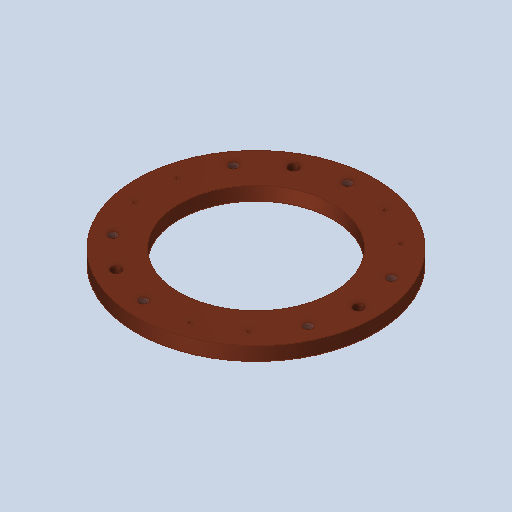
# Autodesk Inventor part: CentralRing-2023-1
Saved by Autodesk Inventor 2026 (Build 300175050, 175E)
## iProperties
Created: 2018-11-20
Part Number: CentralRing-2023-1
Material: Copper
Document SubType Name: Modeling
Designer: schanen
Density: 8.94 g/cm^3
Appearance: Copper - Satin
Mass: 78.801 g
Surface Area: 62.2625 cm^2
Volume: 8.81443 cm^3
Author: schanen
Autodesk Inventor part; units mm, degrees
ref_plane "YZ Plane" through (0, 0, 0) normal (1, 0, 0) x (0, 1, 0)
ref_plane "XZ Plane" through (0, 0, 0) normal (0, 1, 0) x (-1, 0, 0)
ref_plane "XY Plane" through (0, 0, 0) normal (0, 0, 1) x (1, 0, 0)
sketch "Sketch1" plane through (0, 0, 0) normal (1, 0, 0) x (0, 1, 0)
  line L0 (0, 22.5) -> (4, 22.5)
  line L1 (4, 22.5) -> (4, 35)
  line L2 (4, 35) -> (0, 35)
  line L3 (0, 35) -> (0, 22.5)
  line L4 (-0.8, 0) -> (4.8, 0) projected
  point P0 (0, 0)
  dimension "d0" = 22.5
  dimension "d1" = 35
  dimension "d2" = 4
  constraints: 8 end point, 2 parallel, 1 horizontal, 1 perpendicular, 1 point on line
  measures "d0" distance between parallel lines of L4 L0
  measures "d1" distance between parallel lines of L4 L2
  measures "d2" distance of L1.end L2.end
revolve "Revolution1" add sketch "Sketch1" angle 360 about axis through (0, -10, 0) along (0, 1, 0)
sketch "Sketch2" plane through (0, 4, 0) normal (0, 1, 0) x (1, 0, 0)
  point P0 (0, 0)
  point P1 (30, 0)
  dimension "d5" = 30
  measures "d5" distance of point (0, 0) point (30, 0)
hole "Hole1" at (30, 4, 0) direction (0, -1, 0) diameter 3 end through all
pattern_circular "Circular Pattern1" count 3 over 360 about axis through (0, 2, 0) along (0, 1, 0) of "Hole1"
sketch "Sketch3" plane through (0, 4, 0) normal (0, 1, 0) x (1, 0, 0)
  circle A0 centre (0, 0) radius 30 construction
  circle A1 centre (30, 0) radius 1.5 projected
  point P0 (27.4064, 12.2021)
  point P1 (27.4064, -12.2021)
  dimension "d16" = 60
  dimension "d18" = 24
  dimension "d20" = 24
  constraints: 2 point on circle, 1 centre point, 1 coincident
  measures "d16" diameter of A0
hole "Hole2" at (27.4064, 4, -12.2021) at (27.4064, 4, 12.2021) direction (0, -1, 0) diameter 2.6211 end through all thread size "M3x0.35" class "6H" standard "ANSI Metric M Profile"
pattern_circular "Circular Pattern2" count 3 over 360 about axis through (0, 2, 0) along (0, 1, 0) of "Hole2"
sketch "Sketch4" plane through (0, 4, 0) normal (0, 1, 0) x (1, 0, 0)
  circle A0 centre (0, 0) radius 30 construction
  circle A1 centre (27.4064, -12.2021) radius 1.3106 projected
  circle A2 centre (27.4064, 12.2021) radius 1.3106 projected
  point P0 (20.0739, -22.2943)
  point P1 (20.0739, 22.2943)
  dimension "d31" = 60
  dimension "d34" = 24
  dimension "d35" = 24
  constraints: 2 point on circle, 1 centre point, 1 coincident
  measures "d31" diameter of A0
hole "Hole3" at (20.0739, 4, -22.2943) at (20.0739, 4, 22.2943) direction (0, -1, 0) diameter 1 end through all
pattern_circular "Circular Pattern3" count 3 over 360 about axis through (0, 2, 0) along (0, 1, 0) of "Hole3"
body "Solid1"
